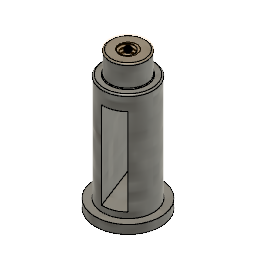
Post (Autodesk Fusion 360 design; units mm, degrees)
Autodesk Fusion 360 part; units mm, degrees
sketch "Sketch1" plane through (0, 0, 0) normal (0, 1, 0) x (1, 0, 0)
  circle A0 centre (0, 0) radius 1.125
  dimension "d1" = 2.25
  measures "d1" diameter of A0
extrude "Extrude1" add sketch "Sketch1" along normal blind 0.3
sketch "Sketch2" plane through (0, 0.3, 0) normal (0, 1, 0) x (-1, 0, 0)
  circle A0 centre (0, 0) radius 1.125
  circle A1 centre (0, 0) radius 0.875
  dimension "d4" = 1.75
  measures "d4" diameter of A1
extrude "Extrude2" add sketch "Sketch2" along normal blind 3.7 contours A1
sketch "Sketch3" plane through (0, 4, 0) normal (0, 1, 0) x (-1, 0, 0)
  circle A0 centre (0, 0) radius 0.875
  circle A1 centre (0, 0) radius 0.625
  dimension "d7" = 1.25
  measures "d7" diameter of A1
extrude "Extrude3" add sketch "Sketch3" along normal blind 0.75 contours A1
ref_plane "WorkPlane1" through (0.3155, 2.7219, 0.8161) normal (0.360602, 0, 0.93272) x (-0.93272, 0, 0.360602)
sketch "Sketch4" plane through (0.3155, 2.7219, 0.8161) normal (0.360602, 0, 0.93272) x (-0.93272, 0, 0.360602)
  line L0 (0.625, -1.2781) -> (-0.625, -1.2781)
  line L1 (0.875, 2.4219) -> (-0.875, 2.4219)
  line L2 (0, -0.7781) -> (-0.35, -0.7781)
  line L3 (-0.35, -0.7781) -> (-0.35, 2.2219)
  line L4 (-0.35, 2.2219) -> (0.35, 2.2219)
  line L5 (0.35, 2.2219) -> (0.35, -0.7781)
  line L6 (0.35, -0.7781) -> (0, -0.7781)
  dimension "d12" = 0.35
extrude "Extrude4" cut sketch "Sketch4" against normal blind 2
sketch "Sketch5" plane through (0, 4.75, 0) normal (0, 1, 0) x (-1, 0, 0)
  circle A0 centre (0, 0) radius 0.625
fillet "Fillet1" radius 0.05 1 edges at (0.8158, 4, -0.3164)
fillet "Fillet2" radius 0.05 1 edges at (0.5827, 4.75, -0.226)
fillet "Fillet3" radius 0.025 1 edges at (0.5827, 4, 0.226)
sketch "Sketch11" plane through (0, 4.75, 0) normal (0, 1, 0) x (-1, 0, 0)
  circle A0 centre (0, 0) radius 0.3
  dimension "d21" = 0.6
  measures "d21" diameter of A0
hole "Hole2" at (0, 4.75, 0) direction (0, -1, 0) diameter 0.6 depth 2.5 tip angle 180
thread "Thread4" "ANSI Metric M Profile 0.55 M0.55x0.125 6H" major diameter 0.5735 minor diameter 0.446 pitch 0.125 angle 60 modelled right hand crest width 0.0156 on face at (0.015, 4.3333, 0.2996) crest through (0, 4.8203, 0.223)
